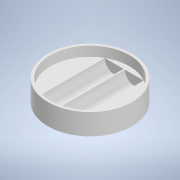
# Autodesk Inventor part: EnclosureBase
Saved by Autodesk Inventor 2020 (Build 240168000, 168)
## iProperties
Created: 2020-10-17
Part Number: EnclosureBase
Material: Generic
Document SubType Name: Modeling
Designer: vmiguel
Density: 1 g/cm^3
Appearance: Default
Author: vmiguel
Autodesk Inventor part; units mm, degrees
ref_plane "YZ Plane" through (0, 0, 0) normal (1, 0, 0) x (0, 1, 0)
ref_plane "XZ Plane" through (0, 0, 0) normal (0, 1, 0) x (-1, 0, 0)
ref_plane "XY Plane" through (0, 0, 0) normal (0, 0, 1) x (1, 0, 0)
sketch "Sketch1" plane through (0, 0, 0) normal (0, 1, 0) x (-1, 0, 0)
  circle A0 centre (0, 0) radius 50
  dimension "d0" = 100
  constraints: 1 centre point, 1 coincident
  measures "d0" diameter of A0
extrude "Extrusion1" add sketch "Sketch1" along normal blind 25
sketch "Sketch2" plane through (0, 0, 0) normal (0, -1, 0) x (1, 0, 0)
  circle A0 centre (0, 0) radius 25.25
  dimension "d3" = 50.5
  constraints: 1 centre point, 1 coincident
  measures "d3" diameter of A0
extrude "Extrusion2" cut sketch "Sketch2" against normal blind 0.4
sketch "Sketch3" plane through (0, 25, 0) normal (0, 1, 0) x (1, 0, 0)
  circle A0 centre (0, 0) radius 47
  circle A1 centre (0, 0) radius 50 projected
  dimension "d6" = 3
  constraints: 1 centre point, 1 coincident
  measures "d6" radial gap between concentric circles of A1 A0
extrude "Extrusion3" cut sketch "Sketch3" against normal blind 11.5 contours A0
sketch "Sketch5" plane through (0, 0, 0) normal (0, 0, 1) x (1, 0, 0)
  line L0 (-47, 13.5) -> (47, 13.5) construction
  circle A0 centre (12, 13.5) radius 11.125
  circle A1 centre (-12, 13.5) radius 11.125
  line L1 (0, 30.15) -> (0, -5.025) construction
  point P0 (0, 0)
  dimension "d9" = 22.25
  dimension "d10" = 22.25
  dimension "d11" = 12
  dimension "d12" = 12
  constraints: 2 centre point, 2 point on line
  measures "d9" diameter of A0
  measures "d10" diameter of A1
  measures "d11" distance from line of L1 A0.centre
  measures "d12" distance from line of A1.centre L1
extrude "Extrusion4" cut sketch "Sketch5" against normal mid plane 81.5
equation "\"d10\" = d9"
equation "\"d12\" = d11"
body "Solid1"
